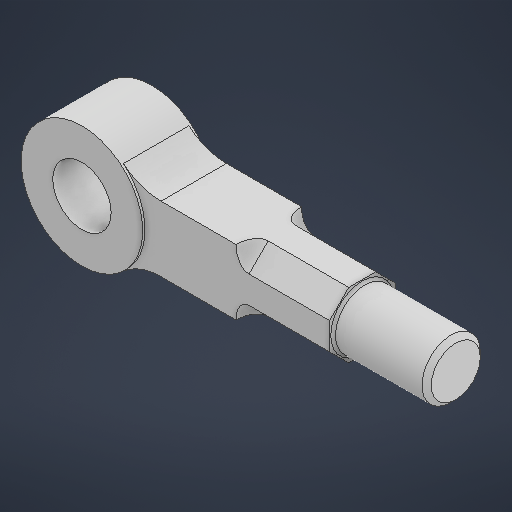
# Autodesk Inventor part: eye-end
Saved by Autodesk Inventor 2026.1 (Build 301233020, 233B)
## iProperties
Created: 2025-12-18
Part Number: eye-end
Material: Generic
Document SubType Name: Modeling
Designer: kngob
Density: 1 g/cm^3
Appearance: Default
Author: kngob
Autodesk Inventor part; units mm, degrees
ref_plane "YZ Plane" through (0, 0, 0) normal (1, 0, 0) x (0, 1, 0)
ref_plane "XZ Plane" through (0, 0, 0) normal (0, 1, 0) x (-1, 0, 0)
ref_plane "XY Plane" through (0, 0, 0) normal (0, 0, 1) x (1, 0, 0)
sketch "Sketch1" plane through (0, 0, 0) normal (0, 0, 1) x (1, 0, 0)
  arc A0 (21.9089, 14) -> (21.9089, -14) centre (0, 0) ccw
  circle A1 centre (0, 0) radius 12.5
  line L0 (21.9089, 14) -> (105, 14)
  line L1 (105, 14) -> (105, -14)
  line L2 (105, -14) -> (21.9089, -14)
  line L3 (-36.8957, 0) -> (84.4086, 0)
  dimension "d0" = 52
  dimension "d1" = 25
  dimension "d2" = 28
  dimension "d3" = 105
  constraints: 8 end point, 2 centre point, 2 coincident, 2 horizontal, 2 point on circle, 1 parallel, 1 perpendicular, 1 other
  measures "d0" diameter of A0
  measures "d1" diameter of A1
  measures "d2" distance of L0.end L1.end
  measures "d3" distance from line of L1 A0.centre
extrude "Extrusion1" add sketch "Sketch1" along normal blind 28
sketch "Sketch2" plane through (0, 0, 28) normal (0, 0, 1) x (1, 0, 0)
  arc A0 (21.9089, 14) -> (21.9089, -14) centre (0, 0) ccw projected
  circle A1 centre (0, 0) radius 26
  circle A2 centre (0, 0) radius 12.5 projected
  point P0 (21.9089, -14)
  constraints: 1 centre point, 1 coincident, 1 concentric
extrude "Extrusion2" add sketch "Sketch2" along normal blind 1
ref_plane "Work Plane1" through (0, 0, 14) normal (0, 0, 1) x (1, 0, 0)
mirror "Mirror2" about plane through (0, 0, 14) normal (0, 0, 1) of "Extrusion2"
sketch "Sketch3" plane through (105, -14, 0) normal (1, 0, 0) x (0, 0, -1)
  circle A0 centre (-14, 14) radius 12.5
  line L0 (0, 0) -> (0, 28) projected
  line L1 (0, 28) -> (-28, 28) projected
  point P0 (0, 14)
  point P1 (0, 14)
  point P2 (-14, 28)
  dimension "d8" = 25
  constraints: 2 midpoint, 1 centre point, 1 horizontal alignment, 1 vertical alignment
  measures "d8" diameter of A0
extrude "Extrusion3" add sketch "Sketch3" along normal blind 40
sketch "Sketch4" plane through (105, -14, 0) normal (1, 0, 0) x (0, 0, -1)
  circle A0 centre (-14, 14) radius 12.5 projected
  line L0 (0, 0) -> (-28, 0) projected
  line L1 (-8.201, 0) -> (-19.799, 0)
  line L2 (-19.799, 0) -> (-28, 8.201)
  line L3 (-28, 8.201) -> (-28, 19.799)
  line L4 (-28, 19.799) -> (-19.799, 28)
  line L5 (-19.799, 28) -> (-8.201, 28)
  line L6 (-8.201, 28) -> (0, 19.799)
  line L7 (0, 19.799) -> (0, 8.201)
  line L8 (0, 8.201) -> (-8.201, 0)
  circle A1 centre (-14, 14) radius 12.5 projected
  line L9 (0, 0) -> (0, 28) projected
  line L10 (0, 28) -> (-28, 28) projected
  line L11 (-28, 0) -> (-28, 28) projected
  line L12 (0, 0) -> (-28, 0) projected
  point P0 (0, 14)
  point P1 (0, 8.201)
  constraints: 16 end point, 1 coincident, 1 point on line, 1 vertical, 17 other
extrude "Extrusion4" cut sketch "Sketch4" against normal blind 40 contours L0 L8 L9 | L0 L11 L2 | L6 L10 L9 | L11 L10 L4
fillet "Fillet1" radius 5.5 4 edges at (65, 9.8995, 23.8995) (65, 9.8995, 4.1005) (65, -9.8995, 4.1005) (65, -9.8995, 23.8995)
fillet "Fillet2" radius 25 2 edges at (21.9089, 14, 14) (21.9089, -14, 14)
fillet "Fillet3" radius 1 1 edges at (105, 0, 26.5)
chamfer "Chamfer1" distance 2 angle 45 1 edges at (145, 0, 26.5)
body "Solid1"
